Autodesk Inventor part; units mm, degrees
(part 2 of 2)
  spline S234 degree 2 poles (-17.2264, -34.5318) (-17.2832, -34.5021) (-17.4906, -34.4503) (-17.6092, -34.4503) knots 0 0 0 1 2 2 2
  spline S235 degree 2 poles (-17.6092, -34.4503) (-17.9896, -34.4503) (-18.4564, -34.964) (-18.5009, -35.4679) knots 0 0 0 1 2 2 2
  spline S236 degree 2 poles (-18.5009, -35.4679) (-18.3552, -35.3666) (-18.0489, -35.2555) (-17.8661, -35.2555) knots 0 0 0 1 2 2 2
  spline S237 degree 2 poles (-17.8661, -35.2555) (-17.6882, -35.2555) (-17.4215, -35.3271) (-17.2758, -35.4358) knots 0 0 0 1 2 2 2
  spline S238 degree 2 poles (-17.2758, -35.4358) (-17.1078, -35.5618) (-16.9448, -35.952) (-16.9448, -36.2139) knots 0 0 0 1 2 2 2
  spline S239 degree 2 poles (-17.3597, -36.2312) (-17.3597, -36.0434) (-17.4585, -35.789) (-17.5672, -35.7001) knots 0 0 0 1 2 2 2
  spline S240 degree 2 poles (-17.5672, -35.7001) (-17.6487, -35.6359) (-17.8513, -35.5939) (-17.9575, -35.5939) knots 0 0 0 1 2 2 2
  spline S241 degree 2 poles (-17.9575, -35.5939) (-18.1007, -35.5939) (-18.37, -35.6803) (-18.5009, -35.7618) knots 0 0 0 1 2 2 2
  spline S242 degree 2 poles (-18.5009, -35.7618) (-18.5034, -35.8063) (-18.5083, -35.8903) (-18.5083, -35.9545) knots 0 0 0 1 2 2 2
  spline S243 degree 2 poles (-18.5083, -35.9545) (-18.5083, -36.2707) (-18.3848, -36.6585) (-18.2909, -36.7597) knots 0 0 0 1 2 2 2
  spline S244 degree 2 poles (-18.2909, -36.7597) (-18.2045, -36.8561) (-18.0168, -36.9326) (-17.9105, -36.9326) knots 0 0 0 1 2 2 2
  spline S245 degree 2 poles (-17.9105, -36.9326) (-17.6635, -36.9326) (-17.3597, -36.5819) (-17.3597, -36.2312) knots 0 0 0 1 2 2 2
  line L293 (-14.8255, -37.2019) -> (-15.2108, -37.2019)
  line L294 (-15.2108, -37.2019) -> (-15.2108, -34.9146)
  line L295 (-15.2108, -34.9146) -> (-14.8255, -34.9146)
  line L296 (-14.8255, -34.9146) -> (-14.8255, -37.2019)
  line L297 (-14.7983, -34.5342) -> (-15.2355, -34.5342)
  line L298 (-15.2355, -34.5342) -> (-15.2355, -34.1341)
  line L299 (-15.2355, -34.1341) -> (-14.7983, -34.1341)
  line L300 (-14.7983, -34.1341) -> (-14.7983, -34.5342)
  line L301 (-12.4642, -37.2019) -> (-12.8495, -37.2019)
  line L302 (-12.8495, -37.2019) -> (-12.8495, -35.8977)
  spline S246 degree 2 poles (-12.8495, -35.8977) (-12.8495, -35.7396) (-12.8791, -35.4679) (-12.9236, -35.3864) knots 0 0 0 1 2 2 2
  spline S247 degree 2 poles (-12.9236, -35.3864) (-12.9705, -35.3) (-13.1385, -35.216) (-13.2817, -35.216) knots 0 0 0 1 2 2 2
  spline S248 degree 2 poles (-13.2817, -35.216) (-13.425, -35.216) (-13.7288, -35.3691) (-13.8745, -35.4926) knots 0 0 0 1 2 2 2
  line L303 (-13.8745, -35.4926) -> (-13.8745, -37.2019)
  line L304 (-13.8745, -37.2019) -> (-14.2599, -37.2019)
  line L305 (-14.2599, -37.2019) -> (-14.2599, -34.9146)
  line L306 (-14.2599, -34.9146) -> (-13.8745, -34.9146)
  line L307 (-13.8745, -34.9146) -> (-13.8745, -35.169)
  spline S249 degree 2 poles (-13.8745, -35.169) (-13.7016, -35.0134) (-13.3682, -34.8504) (-13.1805, -34.8504) knots 0 0 0 1 2 2 2
  spline S250 degree 2 poles (-13.1805, -34.8504) (-12.8445, -34.8504) (-12.4642, -35.295) (-12.4642, -35.7174) knots 0 0 0 1 2 2 2
  line L308 (-12.4642, -35.7174) -> (-12.4642, -37.2019)
  spline S251 degree 2 poles (-11.0143, -37.2537) (-11.2514, -37.2537) (-11.6441, -37.108) (-11.7849, -36.9598) knots 0 0 0 1 2 2 2
  spline S252 degree 2 poles (-11.7849, -36.9598) (-11.9257, -36.8141) (-12.0813, -36.3645) (-12.0813, -36.0632) knots 0 0 0 1 2 2 2
  spline S253 degree 2 poles (-12.0813, -36.0632) (-12.0813, -35.7618) (-11.9208, -35.3222) (-11.7849, -35.174) knots 0 0 0 1 2 2 2
  spline S254 degree 2 poles (-11.7849, -35.174) (-11.6491, -35.0233) (-11.2464, -34.8628) (-11.0143, -34.8628) knots 0 0 0 1 2 2 2
  spline S255 degree 2 poles (-11.0143, -34.8628) (-10.8265, -34.8628) (-10.4758, -34.969) (-10.3399, -35.0381) knots 0 0 0 1 2 2 2
  line L309 (-10.3399, -35.0381) -> (-10.3399, -35.4704)
  line L310 (-10.3399, -35.4704) -> (-10.3622, -35.4704)
  spline S256 degree 2 poles (-10.3622, -35.4704) (-10.4042, -35.4358) (-10.5326, -35.3469) (-10.624, -35.3) knots 0 0 0 1 2 2 2
  spline S257 degree 2 poles (-10.624, -35.3) (-10.7055, -35.2604) (-10.9229, -35.1987) (-11.0217, -35.1987) knots 0 0 0 1 2 2 2
  spline S258 degree 2 poles (-11.0217, -35.1987) (-11.3205, -35.1987) (-11.6836, -35.6507) (-11.6836, -36.0632) knots 0 0 0 1 2 2 2
  spline S259 degree 2 poles (-11.6836, -36.0632) (-11.6836, -36.4658) (-11.3329, -36.9178) (-11.0217, -36.9178) knots 0 0 0 1 2 2 2
  spline S260 degree 2 poles (-11.0217, -36.9178) (-10.834, -36.9178) (-10.4931, -36.7622) (-10.3622, -36.6412) knots 0 0 0 1 2 2 2
  line L311 (-10.3622, -36.6412) -> (-10.3399, -36.6412)
  line L312 (-10.3399, -36.6412) -> (-10.3399, -37.0734)
  spline S261 degree 2 poles (-10.3399, -37.0734) (-10.3968, -37.1006) (-10.5697, -37.1772) (-10.6388, -37.1945) knots 0 0 0 1 2 2 2
  spline S262 degree 2 poles (-10.6388, -37.1945) (-10.7376, -37.2241) (-10.8932, -37.2537) (-11.0143, -37.2537) knots 0 0 0 1 2 2 2
  line L313 (-8.1935, -37.2019) -> (-8.5788, -37.2019)
  line L314 (-8.5788, -37.2019) -> (-8.5788, -35.8977)
  spline S263 degree 2 poles (-8.5788, -35.8977) (-8.5788, -35.7396) (-8.6085, -35.4679) (-8.6529, -35.3864) knots 0 0 0 1 2 2 2
  spline S264 degree 2 poles (-8.6529, -35.3864) (-8.6999, -35.3) (-8.8678, -35.216) (-9.0111, -35.216) knots 0 0 0 1 2 2 2
  spline S265 degree 2 poles (-9.0111, -35.216) (-9.1543, -35.216) (-9.4582, -35.3691) (-9.6039, -35.4926) knots 0 0 0 1 2 2 2
  line L315 (-9.6039, -35.4926) -> (-9.6039, -37.2019)
  line L316 (-9.6039, -37.2019) -> (-9.9892, -37.2019)
  line L317 (-9.9892, -37.2019) -> (-9.9892, -34.018)
  line L318 (-9.9892, -34.018) -> (-9.6039, -34.018)
  line L319 (-9.6039, -34.018) -> (-9.6039, -35.169)
  spline S266 degree 2 poles (-9.6039, -35.169) (-9.431, -35.0134) (-9.0975, -34.8504) (-8.9098, -34.8504) knots 0 0 0 1 2 2 2
  spline S267 degree 2 poles (-8.9098, -34.8504) (-8.5739, -34.8504) (-8.1935, -35.295) (-8.1935, -35.7174) knots 0 0 0 1 2 2 2
  line L320 (-8.1935, -35.7174) -> (-8.1935, -37.2019)
  line L321 (5.3953, -34.6108) -> (4.0763, -37.2019)
  line L322 (4.0763, -37.2019) -> (3.6416, -37.2019)
  line L323 (3.6416, -37.2019) -> (5.0346, -34.512)
  line L324 (5.0346, -34.512) -> (3.4612, -34.512)
  line L325 (3.4612, -34.512) -> (3.4612, -34.1539)
  line L326 (3.4612, -34.1539) -> (5.3953, -34.1539)
  line L327 (5.3953, -34.1539) -> (5.3953, -34.6108)
  line L328 (7.0354, -34.018) -> (5.8423, -37.8638)
  line L329 (5.8423, -37.8638) -> (5.4965, -37.8638)
  line L330 (5.4965, -37.8638) -> (6.6846, -34.018)
  line L331 (6.6846, -34.018) -> (7.0354, -34.018)
  spline S268 degree 2 poles (9.2979, -36.2139) (9.2979, -36.4485) (9.1423, -36.8462) (9.0114, -36.9796) knots 0 0 0 1 2 2 2
  spline S269 degree 2 poles (9.0114, -36.9796) (8.8755, -37.1204) (8.5347, -37.2661) (8.3296, -37.2661) knots 0 0 0 1 2 2 2
  spline S270 degree 2 poles (8.3296, -37.2661) (8.1246, -37.2661) (7.7862, -37.1278) (7.6578, -36.9894) knots 0 0 0 1 2 2 2
  spline S271 degree 2 poles (7.6578, -36.9894) (7.4997, -36.824) (7.3219, -36.2682) (7.3219, -35.8631) knots 0 0 0 1 2 2 2
  spline S272 degree 2 poles (7.3219, -35.8631) (7.3219, -35.4654) (7.4849, -34.8257) (7.6553, -34.5886) knots 0 0 0 1 2 2 2
  spline S273 degree 2 poles (7.6553, -34.5886) (7.8208, -34.3564) (8.3445, -34.0971) (8.6878, -34.0971) knots 0 0 0 1 2 2 2
  spline S274 degree 2 poles (8.6878, -34.0971) (8.7891, -34.0971) (8.9669, -34.1168) (9.0336, -34.139) knots 0 0 0 1 2 2 2
  line L332 (9.0336, -34.139) -> (9.0336, -34.5318)
  line L333 (9.0336, -34.5318) -> (9.0163, -34.5318)
  spline S275 degree 2 poles (9.0163, -34.5318) (8.9595, -34.5021) (8.752, -34.4503) (8.6335, -34.4503) knots 0 0 0 1 2 2 2
  spline S276 degree 2 poles (8.6335, -34.4503) (8.2531, -34.4503) (7.7862, -34.964) (7.7418, -35.4679) knots 0 0 0 1 2 2 2
  spline S277 degree 2 poles (7.7418, -35.4679) (7.8875, -35.3666) (8.1938, -35.2555) (8.3766, -35.2555) knots 0 0 0 1 2 2 2
  spline S278 degree 2 poles (8.3766, -35.2555) (8.5544, -35.2555) (8.8212, -35.3271) (8.9669, -35.4358) knots 0 0 0 1 2 2 2
  spline S279 degree 2 poles (8.9669, -35.4358) (9.1349, -35.5618) (9.2979, -35.952) (9.2979, -36.2139) knots 0 0 0 1 2 2 2
  spline S280 degree 2 poles (8.8829, -36.2312) (8.8829, -36.0434) (8.7841, -35.789) (8.6754, -35.7001) knots 0 0 0 1 2 2 2
  spline S281 degree 2 poles (8.6754, -35.7001) (8.5939, -35.6359) (8.3914, -35.5939) (8.2852, -35.5939) knots 0 0 0 1 2 2 2
  spline S282 degree 2 poles (8.2852, -35.5939) (8.1419, -35.5939) (7.8727, -35.6803) (7.7418, -35.7618) knots 0 0 0 1 2 2 2
  spline S283 degree 2 poles (7.7418, -35.7618) (7.7393, -35.8063) (7.7344, -35.8903) (7.7344, -35.9545) knots 0 0 0 1 2 2 2
  spline S284 degree 2 poles (7.7344, -35.9545) (7.7344, -36.2707) (7.8579, -36.6585) (7.9517, -36.7597) knots 0 0 0 1 2 2 2
  spline S285 degree 2 poles (7.9517, -36.7597) (8.0382, -36.8561) (8.2259, -36.9326) (8.3321, -36.9326) knots 0 0 0 1 2 2 2
  spline S286 degree 2 poles (8.3321, -36.9326) (8.5791, -36.9326) (8.8829, -36.5819) (8.8829, -36.2312) knots 0 0 0 1 2 2 2
  line L334 (11.4172, -37.2019) -> (11.0318, -37.2019)
  line L335 (11.0318, -37.2019) -> (11.0318, -34.9146)
  line L336 (11.0318, -34.9146) -> (11.4172, -34.9146)
  line L337 (11.4172, -34.9146) -> (11.4172, -37.2019)
  line L338 (11.4443, -34.5342) -> (11.0071, -34.5342)
  line L339 (11.0071, -34.5342) -> (11.0071, -34.1341)
  line L340 (11.0071, -34.1341) -> (11.4443, -34.1341)
  line L341 (11.4443, -34.1341) -> (11.4443, -34.5342)
  line L342 (13.7785, -37.2019) -> (13.3932, -37.2019)
  line L343 (13.3932, -37.2019) -> (13.3932, -35.8977)
  spline S287 degree 2 poles (13.3932, -35.8977) (13.3932, -35.7396) (13.3635, -35.4679) (13.3191, -35.3864) knots 0 0 0 1 2 2 2
  spline S288 degree 2 poles (13.3191, -35.3864) (13.2721, -35.3) (13.1042, -35.216) (12.9609, -35.216) knots 0 0 0 1 2 2 2
  spline S289 degree 2 poles (12.9609, -35.216) (12.8177, -35.216) (12.5139, -35.3691) (12.3681, -35.4926) knots 0 0 0 1 2 2 2
  line L344 (12.3681, -35.4926) -> (12.3681, -37.2019)
  line L345 (12.3681, -37.2019) -> (11.9828, -37.2019)
  line L346 (11.9828, -37.2019) -> (11.9828, -34.9146)
  line L347 (11.9828, -34.9146) -> (12.3681, -34.9146)
  line L348 (12.3681, -34.9146) -> (12.3681, -35.169)
  spline S290 degree 2 poles (12.3681, -35.169) (12.541, -35.0134) (12.8745, -34.8504) (13.0622, -34.8504) knots 0 0 0 1 2 2 2
  spline S291 degree 2 poles (13.0622, -34.8504) (13.3981, -34.8504) (13.7785, -35.295) (13.7785, -35.7174) knots 0 0 0 1 2 2 2
  line L349 (13.7785, -35.7174) -> (13.7785, -37.2019)
  spline S292 degree 2 poles (15.2284, -37.2537) (14.9913, -37.2537) (14.5985, -37.108) (14.4578, -36.9598) knots 0 0 0 1 2 2 2
  spline S293 degree 2 poles (14.4578, -36.9598) (14.317, -36.8141) (14.1614, -36.3645) (14.1614, -36.0632) knots 0 0 0 1 2 2 2
  spline S294 degree 2 poles (14.1614, -36.0632) (14.1614, -35.7618) (14.3219, -35.3222) (14.4578, -35.174) knots 0 0 0 1 2 2 2
  spline S295 degree 2 poles (14.4578, -35.174) (14.5936, -35.0233) (14.9962, -34.8628) (15.2284, -34.8628) knots 0 0 0 1 2 2 2
  spline S296 degree 2 poles (15.2284, -34.8628) (15.4161, -34.8628) (15.7669, -34.969) (15.9027, -35.0381) knots 0 0 0 1 2 2 2
  line L350 (15.9027, -35.0381) -> (15.9027, -35.4704)
  line L351 (15.9027, -35.4704) -> (15.8805, -35.4704)
  spline S297 degree 2 poles (15.8805, -35.4704) (15.8385, -35.4358) (15.7101, -35.3469) (15.6187, -35.3) knots 0 0 0 1 2 2 2
  spline S298 degree 2 poles (15.6187, -35.3) (15.5372, -35.2604) (15.3198, -35.1987) (15.221, -35.1987) knots 0 0 0 1 2 2 2
  spline S299 degree 2 poles (15.221, -35.1987) (14.9221, -35.1987) (14.559, -35.6507) (14.559, -36.0632) knots 0 0 0 1 2 2 2
  spline S300 degree 2 poles (14.559, -36.0632) (14.559, -36.4658) (14.9098, -36.9178) (15.221, -36.9178) knots 0 0 0 1 2 2 2
  spline S301 degree 2 poles (15.221, -36.9178) (15.4087, -36.9178) (15.7496, -36.7622) (15.8805, -36.6412) knots 0 0 0 1 2 2 2
  line L352 (15.8805, -36.6412) -> (15.9027, -36.6412)
  line L353 (15.9027, -36.6412) -> (15.9027, -37.0734)
  spline S302 degree 2 poles (15.9027, -37.0734) (15.8459, -37.1006) (15.673, -37.1772) (15.6038, -37.1945) knots 0 0 0 1 2 2 2
  spline S303 degree 2 poles (15.6038, -37.1945) (15.505, -37.2241) (15.3494, -37.2537) (15.2284, -37.2537) knots 0 0 0 1 2 2 2
  line L354 (18.0492, -37.2019) -> (17.6638, -37.2019)
  line L355 (17.6638, -37.2019) -> (17.6638, -35.8977)
  spline S304 degree 2 poles (17.6638, -35.8977) (17.6638, -35.7396) (17.6342, -35.4679) (17.5897, -35.3864) knots 0 0 0 1 2 2 2
  spline S305 degree 2 poles (17.5897, -35.3864) (17.5428, -35.3) (17.3748, -35.216) (17.2316, -35.216) knots 0 0 0 1 2 2 2
  spline S306 degree 2 poles (17.2316, -35.216) (17.0883, -35.216) (16.7845, -35.3691) (16.6388, -35.4926) knots 0 0 0 1 2 2 2
  line L356 (16.6388, -35.4926) -> (16.6388, -37.2019)
  line L357 (16.6388, -37.2019) -> (16.2535, -37.2019)
  line L358 (16.2535, -37.2019) -> (16.2535, -34.018)
  line L359 (16.2535, -34.018) -> (16.6388, -34.018)
  line L360 (16.6388, -34.018) -> (16.6388, -35.169)
  spline S307 degree 2 poles (16.6388, -35.169) (16.8117, -35.0134) (17.1451, -34.8504) (17.3329, -34.8504) knots 0 0 0 1 2 2 2
  spline S308 degree 2 poles (17.3329, -34.8504) (17.6688, -34.8504) (18.0492, -35.295) (18.0492, -35.7174) knots 0 0 0 1 2 2 2
  line L361 (18.0492, -35.7174) -> (18.0492, -37.2019)
  spline S309 degree 2 poles (33.5948, -34.4429) (33.4836, -34.4429) (33.2638, -34.4972) (33.1576, -34.5392) knots 0 0 0 1 2 2 2
  spline S310 degree 2 poles (33.1576, -34.5392) (33.0588, -34.5812) (32.9131, -34.6701) (32.8563, -34.7096) knots 0 0 0 1 2 2 2
  line L362 (32.8563, -34.7096) -> (32.8316, -34.7096)
  line L363 (32.8316, -34.7096) -> (32.8316, -34.2774)
  spline S311 degree 2 poles (32.8316, -34.2774) (32.9649, -34.2057) (33.4219, -34.0896) (33.6269, -34.0896) knots 0 0 0 1 2 2 2
  spline S312 degree 2 poles (33.6269, -34.0896) (33.8344, -34.0896) (34.1431, -34.1736) (34.2691, -34.2625) knots 0 0 0 1 2 2 2
  spline S313 degree 2 poles (34.2691, -34.2625) (34.4025, -34.3589) (34.5408, -34.638) (34.5408, -34.8257) knots 0 0 0 1 2 2 2
  spline S314 degree 2 poles (34.5408, -34.8257) (34.5408, -35.0777) (34.2098, -35.458) (33.9776, -35.5074) knots 0 0 0 1 2 2 2
  line L364 (33.9776, -35.5074) -> (33.9776, -35.5371)
  spline S315 degree 2 poles (33.9776, -35.5371) (34.074, -35.5568) (34.2938, -35.6458) (34.3877, -35.7347) knots 0 0 0 1 2 2 2
  spline S316 degree 2 poles (34.3877, -35.7347) (34.4815, -35.8211) (34.6001, -36.0978) (34.6001, -36.2978) knots 0 0 0 1 2 2 2
  spline S317 degree 2 poles (34.6001, -36.2978) (34.6001, -36.5029) (34.4593, -36.8511) (34.3309, -36.9845) knots 0 0 0 1 2 2 2
  spline S318 degree 2 poles (34.3309, -36.9845) (34.1975, -37.1228) (33.8196, -37.2661) (33.58, -37.2661) knots 0 0 0 1 2 2 2
  spline S319 degree 2 poles (33.58, -37.2661) (33.3503, -37.2661) (32.9007, -37.1549) (32.7476, -37.0784) knots 0 0 0 1 2 2 2
  line L365 (32.7476, -37.0784) -> (32.7476, -36.6461)
  line L366 (32.7476, -36.6461) -> (32.7772, -36.6461)
  spline S320 degree 2 poles (32.7772, -36.6461) (32.9057, -36.74) (33.3404, -36.9129) (33.5553, -36.9129) knots 0 0 0 1 2 2 2
  spline S321 degree 2 poles (33.5553, -36.9129) (33.6812, -36.9129) (33.9332, -36.8338) (34.0172, -36.7424) knots 0 0 0 1 2 2 2
  spline S322 degree 2 poles (34.0172, -36.7424) (34.0987, -36.6511) (34.1851, -36.4337) (34.1851, -36.2682) knots 0 0 0 1 2 2 2
  spline S323 degree 2 poles (34.1851, -36.2682) (34.1851, -36.1027) (34.0888, -35.8878) (34.0023, -35.8261) knots 0 0 0 1 2 2 2
  spline S324 degree 2 poles (34.0023, -35.8261) (33.9159, -35.7643) (33.6812, -35.7174) (33.5429, -35.7174) knots 0 0 0 1 2 2 2
  line L367 (33.5429, -35.7174) -> (33.37, -35.7174)
  line L368 (33.37, -35.7174) -> (33.37, -35.379)
  line L369 (33.37, -35.379) -> (33.5059, -35.379)
  spline S325 degree 2 poles (33.5059, -35.379) (33.78, -35.379) (34.1259, -35.1172) (34.1259, -34.8677) knots 0 0 0 1 2 2 2
  spline S326 degree 2 poles (34.1259, -34.8677) (34.1259, -34.7516) (34.0369, -34.5861) (33.9653, -34.5367) knots 0 0 0 1 2 2 2
  spline S327 degree 2 poles (33.9653, -34.5367) (33.8887, -34.4848) (33.701, -34.4429) (33.5948, -34.4429) knots 0 0 0 1 2 2 2
  line L370 (36.3266, -34.018) -> (35.1336, -37.8638)
  line L371 (35.1336, -37.8638) -> (34.7878, -37.8638)
  line L372 (34.7878, -37.8638) -> (35.9759, -34.018)
  line L373 (35.9759, -34.018) -> (36.3266, -34.018)
  spline S328 degree 2 poles (37.5839, -37.271) (37.3566, -37.271) (36.9837, -37.1352) (36.8527, -37.0092) knots 0 0 0 1 2 2 2
  spline S329 degree 2 poles (36.8527, -37.0092) (36.7243, -36.8857) (36.5909, -36.5498) (36.5909, -36.3596) knots 0 0 0 1 2 2 2
  spline S330 degree 2 poles (36.5909, -36.3596) (36.5909, -36.1126) (36.8552, -35.6976) (37.1072, -35.5741) knots 0 0 0 1 2 2 2
  line L374 (37.1072, -35.5741) -> (37.1072, -35.5618)
  spline S331 degree 2 poles (37.1072, -35.5618) (36.8824, -35.4309) (36.665, -35.1196) (36.665, -34.8875) knots 0 0 0 1 2 2 2
  spline S332 degree 2 poles (36.665, -34.8875) (36.665, -34.5441) (37.1837, -34.0847) (37.5839, -34.0847) knots 0 0 0 1 2 2 2
  spline S333 degree 2 poles (37.5839, -34.0847) (37.9988, -34.0847) (38.5002, -34.5194) (38.5002, -34.8603) knots 0 0 0 1 2 2 2
  spline S334 degree 2 poles (38.5002, -34.8603) (38.5002, -35.0653) (38.2607, -35.4654) (38.0359, -35.5791) knots 0 0 0 1 2 2 2
  line L375 (38.0359, -35.5791) -> (38.0359, -35.5914)
  spline S335 degree 2 poles (38.0359, -35.5914) (38.3026, -35.7149) (38.5768, -36.0706) (38.5768, -36.3522) knots 0 0 0 1 2 2 2
  spline S336 degree 2 poles (38.5768, -36.3522) (38.5768, -36.7424) (38.0087, -37.271) (37.5839, -37.271) knots 0 0 0 1 2 2 2
  spline S337 degree 2 poles (38.1569, -36.3917) (38.1569, -36.204) (38.0087, -35.9817) (37.7988, -35.8681) knots 0 0 0 1 2 2 2
  spline S338 degree 2 poles (37.7988, -35.8681) (37.7296, -35.8285) (37.4974, -35.7371) (37.3517, -35.6779) knots 0 0 0 1 2 2 2
  spline S339 degree 2 poles (37.3517, -35.6779) (37.1837, -35.789) (37.0034, -36.12) (37.0034, -36.33) knots 0 0 0 1 2 2 2
  spline S340 degree 2 poles (37.0034, -36.33) (37.0034, -36.6066) (37.3369, -36.9672) (37.5888, -36.9672) knots 0 0 0 1 2 2 2
  spline S341 degree 2 poles (37.5888, -36.9672) (37.8457, -36.9672) (38.1569, -36.6585) (38.1569, -36.3917) knots 0 0 0 1 2 2 2
  spline S342 degree 2 poles (38.1001, -34.8652) (38.1001, -34.6602) (37.8259, -34.386) (37.5814, -34.386) knots 0 0 0 1 2 2 2
  spline S343 degree 2 poles (37.5814, -34.386) (37.3591, -34.386) (37.0751, -34.6306) (37.0751, -34.8405) knots 0 0 0 1 2 2 2
  spline S344 degree 2 poles (37.0751, -34.8405) (37.0751, -34.9912) (37.2208, -35.2012) (37.3665, -35.2851) knots 0 0 0 1 2 2 2
  spline S345 degree 2 poles (37.3665, -35.2851) (37.4283, -35.3197) (37.6901, -35.4407) (37.7963, -35.4753) knots 0 0 0 1 2 2 2
  spline S346 degree 2 poles (37.7963, -35.4753) (37.9741, -35.3395) (38.1001, -35.0505) (38.1001, -34.8652) knots 0 0 0 1 2 2 2
  line L376 (40.7084, -37.2019) -> (40.3231, -37.2019)
  line L377 (40.3231, -37.2019) -> (40.3231, -34.9146)
  line L378 (40.3231, -34.9146) -> (40.7084, -34.9146)
  line L379 (40.7084, -34.9146) -> (40.7084, -37.2019)
  line L380 (40.7356, -34.5342) -> (40.2984, -34.5342)
  line L381 (40.2984, -34.5342) -> (40.2984, -34.1341)
  line L382 (40.2984, -34.1341) -> (40.7356, -34.1341)
  line L383 (40.7356, -34.1341) -> (40.7356, -34.5342)
  line L384 (43.0698, -37.2019) -> (42.6845, -37.2019)
  line L385 (42.6845, -37.2019) -> (42.6845, -35.8977)
  spline S347 degree 2 poles (42.6845, -35.8977) (42.6845, -35.7396) (42.6548, -35.4679) (42.6104, -35.3864) knots 0 0 0 1 2 2 2
  spline S348 degree 2 poles (42.6104, -35.3864) (42.5634, -35.3) (42.3955, -35.216) (42.2522, -35.216) knots 0 0 0 1 2 2 2
  spline S349 degree 2 poles (42.2522, -35.216) (42.1089, -35.216) (41.8051, -35.3691) (41.6594, -35.4926) knots 0 0 0 1 2 2 2
  line L386 (41.6594, -35.4926) -> (41.6594, -37.2019)
  line L387 (41.6594, -37.2019) -> (41.2741, -37.2019)
  line L388 (41.2741, -37.2019) -> (41.2741, -34.9146)
  line L389 (41.2741, -34.9146) -> (41.6594, -34.9146)
  line L390 (41.6594, -34.9146) -> (41.6594, -35.169)
  spline S350 degree 2 poles (41.6594, -35.169) (41.8323, -35.0134) (42.1658, -34.8504) (42.3535, -34.8504) knots 0 0 0 1 2 2 2
  spline S351 degree 2 poles (42.3535, -34.8504) (42.6894, -34.8504) (43.0698, -35.295) (43.0698, -35.7174) knots 0 0 0 1 2 2 2
  line L391 (43.0698, -35.7174) -> (43.0698, -37.2019)
  spline S352 degree 2 poles (44.5197, -37.2537) (44.2826, -37.2537) (43.8898, -37.108) (43.749, -36.9598) knots 0 0 0 1 2 2 2
  spline S353 degree 2 poles (43.749, -36.9598) (43.6082, -36.8141) (43.4526, -36.3645) (43.4526, -36.0632) knots 0 0 0 1 2 2 2
  spline S354 degree 2 poles (43.4526, -36.0632) (43.4526, -35.7618) (43.6132, -35.3222) (43.749, -35.174) knots 0 0 0 1 2 2 2
  spline S355 degree 2 poles (43.749, -35.174) (43.8849, -35.0233) (44.2875, -34.8628) (44.5197, -34.8628) knots 0 0 0 1 2 2 2
  spline S356 degree 2 poles (44.5197, -34.8628) (44.7074, -34.8628) (45.0581, -34.969) (45.194, -35.0381) knots 0 0 0 1 2 2 2
  line L392 (45.194, -35.0381) -> (45.194, -35.4704)
  line L393 (45.194, -35.4704) -> (45.1718, -35.4704)
  spline S357 degree 2 poles (45.1718, -35.4704) (45.1298, -35.4358) (45.0013, -35.3469) (44.9099, -35.3) knots 0 0 0 1 2 2 2
  spline S358 degree 2 poles (44.9099, -35.3) (44.8284, -35.2604) (44.6111, -35.1987) (44.5123, -35.1987) knots 0 0 0 1 2 2 2
  spline S359 degree 2 poles (44.5123, -35.1987) (44.2134, -35.1987) (43.8503, -35.6507) (43.8503, -36.0632) knots 0 0 0 1 2 2 2
  spline S360 degree 2 poles (43.8503, -36.0632) (43.8503, -36.4658) (44.201, -36.9178) (44.5123, -36.9178) knots 0 0 0 1 2 2 2
  spline S361 degree 2 poles (44.5123, -36.9178) (44.7, -36.9178) (45.0409, -36.7622) (45.1718, -36.6412) knots 0 0 0 1 2 2 2
  line L394 (45.1718, -36.6412) -> (45.194, -36.6412)
  line L395 (45.194, -36.6412) -> (45.194, -37.0734)
  spline S362 degree 2 poles (45.194, -37.0734) (45.1372, -37.1006) (44.9643, -37.1772) (44.8951, -37.1945) knots 0 0 0 1 2 2 2
  spline S363 degree 2 poles (44.8951, -37.1945) (44.7963, -37.2241) (44.6407, -37.2537) (44.5197, -37.2537) knots 0 0 0 1 2 2 2
  line L396 (47.3404, -37.2019) -> (46.9551, -37.2019)
  line L397 (46.9551, -37.2019) -> (46.9551, -35.8977)
  spline S364 degree 2 poles (46.9551, -35.8977) (46.9551, -35.7396) (46.9255, -35.4679) (46.881, -35.3864) knots 0 0 0 1 2 2 2
  spline S365 degree 2 poles (46.881, -35.3864) (46.8341, -35.3) (46.6661, -35.216) (46.5229, -35.216) knots 0 0 0 1 2 2 2
  spline S366 degree 2 poles (46.5229, -35.216) (46.3796, -35.216) (46.0758, -35.3691) (45.9301, -35.4926) knots 0 0 0 1 2 2 2
  line L398 (45.9301, -35.4926) -> (45.9301, -37.2019)
  line L399 (45.9301, -37.2019) -> (45.5447, -37.2019)
  line L400 (45.5447, -37.2019) -> (45.5447, -34.018)
  line L401 (45.5447, -34.018) -> (45.9301, -34.018)
  line L402 (45.9301, -34.018) -> (45.9301, -35.169)
  spline S367 degree 2 poles (45.9301, -35.169) (46.103, -35.0134) (46.4364, -34.8504) (46.6241, -34.8504) knots 0 0 0 1 2 2 2
  spline S368 degree 2 poles (46.6241, -34.8504) (46.9601, -34.8504) (47.3404, -35.295) (47.3404, -35.7174) knots 0 0 0 1 2 2 2
  line L403 (47.3404, -35.7174) -> (47.3404, -37.2019)
  point P0 (0, 0)
  dimension "d45" = 8.7721
  dimension "d46" = 40.64
  dimension "d50" = 90
  dimension "d52" = 90
  dimension "d53" = 90
  dimension "d54" = 90
  dimension "d55" = 90
  dimension "d56" = 90
  constraints: 48 end point, 15 horizontal, 14 point on circle, 7 parallel, 3 collinear, 3 tangent, 2 perpendicular, 2 vertical, 1 horizontal alignment, 1 other
  measures "d45" distance between parallel lines of L1 L0
  measures "d46" distance between parallel lines of L5 L0
  measures "d50" angle of L9 L2
  measures "d52" angle of L11 L1
  measures "d53" angle of L13 L3
  measures "d54" angle of L15 L4
  measures "d55" angle of L19 L6
  measures "d56" angle of L21 L7
extrude "textLabels" cut sketch "Sketch7" against normal blind 2.3813
fillet "Fillet1" radius 3.175 8 edges at (-53.7972, 0, -12.7) (-28.3464, 0, -12.7) (1.4224, 0, -12.7) (30.9372, 0, -12.7) (33.3451, 0, 19.05) (4.9428, 0, 19.05) (-21.4274, 0, 19.05) (-46.7817, 0, 19.05)
fillet "Fillet2" radius 3.175 4 edges at (-63.5, -3.175, 44.45) (-63.5, -3.175, -44.45) (63.5, -3.175, 44.45) (63.5, -3.175, -44.45)
equation "\"gap0\" = frontGapBetweenHoles"
equation "\"gap1\" = 0.5 * hex5_16inchHole + 0.5 * hex1_4inchHole + frontGapBetweenHoles"
equation "\"gap2\" = 0.5 * hex3_8inchHole + 0.5 * hex5_16inchHole + frontGapBetweenHoles"
equation "\"gap3\" = 0.5 * hex7_16inchHole + 0.5 * hex3_8inchHole + frontGapBetweenHoles"
equation "\"gap5\" = backGapBetweenHoles"
equation "\"gap6\" = 0.5 * hex9_16inchHole + 0.5 * hex1_2inchHole + backGapBetweenHoles"
equation "\"gap7\" = 0.5 * hex5_8inchHole + 0.5 * hex9_16inchHole + backGapBetweenHoles"
equation "\"gap8\" = 0.5 * hex3_4inchHole + 0.5 * hex5_8inchHole + backGapBetweenHoles"
equation "\"d46\" = centerLineForBackText"
equation "\"frontGapBetweenHoles\" = 16.71828"
equation "\"backGapBetweenHoles\" = 9.7028"
equation "\"centerLineForFrontText\" = 8.3185"
equation "\"centerLineForBackText\" = 40.64"
body "Solid1"
